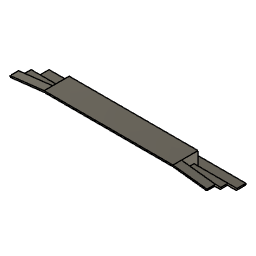
Weichenabdeckung_2Weg_1_v4 (Autodesk Fusion 360 design; units mm, degrees)
Autodesk Fusion 360 part; units mm, degrees
note: some values were not read from the file. Set by a fixed rule: which face or edge a step refers to.
sketch "Skizze1" plane through (0, 0, 0) normal (1, 0, 0) x (0, 1, 0)
  line L0 (0, 0) -> (0, 1.3575)
  line L1 (0, 1.3575) -> (0, 8.8)
  line L2 (0, 8.8) -> (4.75, 8.8)
  line L3 (4.75, 8.8) -> (7.75, 5.8)
  line L4 (7.75, 5.8) -> (11.75, 5.8)
  line L5 (11.75, 5.8) -> (16.75, 0.8)
  line L6 (16.75, 0.8) -> (21.75, 0.8)
  line L7 (21.75, 0.8) -> (21.75, 0)
  line L8 (21.75, 0) -> (0, 0)
  dimension "d1" = 4.75
  dimension "d2" = 3
  dimension "d3" = 3
  dimension "d4" = 4
  dimension "d5" = 5
  dimension "d6" = 5
  dimension "d7" = 0.8
  dimension "d8" = 5
  constraint coincident L0.start L8.end
  constraint vertical L0
  constraint parallel L0 L1
  constraint perpendicular L1 L2
  constraint perpendicular L1 L4
  constraint parallel L4 L6
  constraint perpendicular L6 L7
  constraint horizontal L8
  measures "d1" distance of L1.end L2.end
  measures "d2" horizontal distance of L2.end L3.end
  measures "d3" vertical distance of L2.end L3.end
  measures "d4" distance of L3.end L4.end
  measures "d5" horizontal distance of L4.end L5.end
  measures "d6" vertical distance of L4.end L5.end
  measures "d7" distance of L6.end L7.end
  measures "d8" distance of L5.end L6.end
extrude "Extrusion1" add sketch "Skizze1" along normal blind 110
sketch "Skizze2" plane through (0, 0, 8.8) normal (0, 0, 1) x (-1, 0, 0)
  line L0 (0, -4.75) -> (0, 0)
  line L1 (0, 0) -> (-110, 0)
  line L2 (-110, 0) -> (-110, -4.75)
  line L3 (-110, -4.75) -> (0, -4.75)
  line L4 (-19, 0) -> (-19, -9)
  line L5 (-19, -9) -> (-37, -14)
  line L6 (-37, -14) -> (-73, -14)
  line L7 (-73, -14) -> (-91, -9)
  line L8 (-91, 0) -> (-91, -9)
  line L9 (-19, 0) -> (0, 0) construction
  line L10 (-91, 0) -> (-110, 0) construction
  dimension "d11" = 72
  dimension "d12" = 14
  dimension "d13" = 36
  dimension "d14" = 9
  constraint coincident L1 L4.start
  constraint perpendicular L3 L4
  constraint perpendicular L4 L6
  constraint coincident L1 L8.start
  constraint perpendicular L3 L8
  constraint coincident L0.end L1.start
  constraint coincident L1.end L2.start
  constraint equal L9 L10
  constraint equal L4 L8
  constraint equal L5 L7
  measures "d11" distance of L4.start L8.start
  measures "d12" distance of L1 L6
  measures "d13" distance of L5.end L6.end
  measures "d14" distance of L4.start L4.end
extrude "Extrusion2" add sketch "Skizze2" along normal blind 2.2 and the other way up to surface (8 mm away) contours L3 L4 L5 L6 L7 L8 | L1 L3 L4 L8
sketch "Skizze3" plane through (0, 0, 0) normal (0, -1, 0) x (1, 0, 0)
  line L0 (19, 8.8) -> (0, 8.8)
  line L1 (0, 8.8) -> (0, 0)
  line L2 (0, 0) -> (110, 0)
  line L3 (110, 0) -> (110, 8.8)
  line L4 (110, 8.8) -> (91, 8.8)
  line L5 (91, 8.8) -> (91, 11)
  line L6 (91, 11) -> (19, 11)
  line L7 (19, 11) -> (19, 8.8)
  line L8 (91, 11) -> (110, 8.8)
  line L9 (91, 11) -> (103.2214, 8.8)
  constraint coincident L5.end L6.start
  constraint coincident L3.end L4.start
  constraint coincident L4 L9.end
ref_plane "Arbeitsebene1" through (55, 4.5, 8.4) normal (1, 0, 0) x (0, 1, 0)
extrude "Extrusion3" add sketch "Skizze3" against normal blind 4.75 contours L4 L5 L9 | L4 L8 L9
mirror "Spiegeln2" about plane through (55, 4.5, 8.4) normal (1, 0, 0) of "Extrusion3"
sketch "Skizze4" plane through (0, 0, 11) normal (0, 0, 1) x (-1, 0, 0)
  line L0 (-19, 0) -> (-91, 0)
  line L1 (-91, 0) -> (-91, -4.75)
  line L2 (-91, -4.75) -> (-91, -9)
  line L3 (-91, -9) -> (-73, -14)
  line L4 (-73, -14) -> (-37, -14)
  line L5 (-37, -14) -> (-19, -9)
  line L6 (-19, -9) -> (-19, -4.75)
  line L7 (-19, -4.75) -> (-19, 0)
  line L8 (-91, 0) -> (-19, 0)
  line L9 (-19, 0) -> (-19, -14)
  line L10 (-19, -14) -> (-91, -14)
  line L11 (-91, -14) -> (-91, 0)
  constraint horizontal L8
  constraint vertical L9
  constraint horizontal L10
  constraint vertical L11
  constraint coincident L0.end L1.start
  constraint collinear L7 L9
  constraint collinear L4 L10
extrude "Extrusion7" add sketch "Skizze4" against normal through all of body 1 contours L5 L9 L10 | L3 L10 L11
shell "Schale1" thickness 0.8 removed faces 1 at (36.6667, 14.5, 0)
extrude "Extrusion4" cut 1 faces at (66.9846, 0.8, 3.4) along direction (0, -1, 0) through all
extrude "Extrusion5" cut 1 faces at (109.2, 7.9458, 1.6667) along direction (1, 0, 0) through all
extrude "Extrusion6" cut 1 faces at (0.8, 7.9458, 1.6667) along direction (-1, 0, 0) through all
